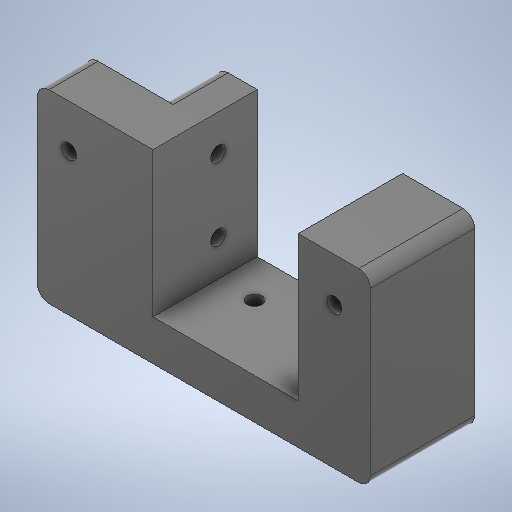
# Autodesk Inventor part: lift_encoder_frame
Saved by Autodesk Inventor 2026.2 (Build 302298010, 298A)
## iProperties
Created: 2026-05-19
Part Number: lift_encoder_frame
Material: ABS Plastic
Document SubType Name: Modeling
Designer: chanh
Density: 1.06 g/cm^3
Appearance: Smooth - White
Author: chanh
Autodesk Inventor part; units mm, degrees
note: some values were not read from the file. Chosen so that the rebuilt part matches the saved one: direction of "Hole3".
ref_plane "YZ Plane" through (0, 0, 0) normal (1, 0, 0) x (0, 1, 0)
ref_plane "XZ Plane" through (0, 0, 0) normal (0, 1, 0) x (-1, 0, 0)
ref_plane "XY Plane" through (0, 0, 0) normal (0, 0, 1) x (1, 0, 0)
sketch "Sketch1" plane through (0, 0, 0) normal (0, 0, 1) x (1, 0, 0)
  line L0 (-50, -64) -> (50, -64)
  line L1 (50, -64) -> (50, 0)
  line L2 (50, 0) -> (-50, 0)
  line L3 (-50, 0) -> (-50, -64)
  line L4 (-50, -64) -> (50, 0) construction
  line L5 (50, -64) -> (-50, 0) construction
  line L6 (-25.1, -50) -> (25.1, -50)
  line L7 (25.1, -50) -> (25.1, 0)
  line L8 (25.1, 0) -> (-25.1, 0)
  line L9 (-25.1, 0) -> (-25.1, -50)
  line L10 (-25.1, -50) -> (25.1, 0) construction
  line L11 (25.1, -50) -> (-25.1, 0) construction
  point P0 (0, 0)
  point P1 (0, -32)
  point P2 (0, 0)
  point P3 (0, -25)
  point P4 (-25.1, 0)
  dimension "d0" = 100
  dimension "d1" = 64
  dimension "d2" = 50.2
  dimension "d3" = 50
  constraints: 24 end point, 6 midpoint, 4 parallel, 2 horizontal, 2 perpendicular, 1 coincident, 1 point on line
  measures "d0" distance of L1.end L2.end
  measures "d1" distance between parallel lines of L2 L0
  measures "d2" distance between parallel lines of L7 L9
  measures "d3" distance between parallel lines of L2 L6
extrude "Extrusion1" add sketch "Sketch1" along normal blind 36 contours L3 L2 L9 L6 L7 L1 L0
sketch "Sketch2" plane through (0, 0, 0) normal (0, 0, -1) x (-1, 0, 0)
  line L0 (-50, 0) -> (-25.1, 0) projected
  line L1 (-25.1, 0) -> (-25.1, -50) projected
  line L2 (-25.1, -50) -> (25.1, -50) projected
  line L3 (25.1, -50) -> (25.1, 0) projected
  line L4 (25.1, 0) -> (50, 0) projected
  line L5 (50, 0) -> (50, -64) projected
  line L6 (50, -64) -> (-50, -64) projected
  line L7 (-50, -64) -> (-50, 0) projected
  line L8 (25.1, 0) -> (50, 0)
  line L9 (50, 0) -> (50, -50)
  line L10 (50, -50) -> (25.1, -50)
  line L11 (25.1, -50) -> (25.1, 0)
  point P0 (0, 0)
  point P1 (25.1, -50)
  constraints: 8 end point, 2 parallel, 1 collinear, 1 horizontal, 1 perpendicular, 1 point on line
extrude "Extrusion2" cut sketch "Sketch2" against normal blind 19 contours L3 L4 L5 L10
sketch "Sketch3" plane through (-50, -64, 0) normal (-1, 0, 0) x (0, 0, 1)
  line L0 (19, 64) -> (19, 14) projected
  line L1 (19, 14) -> (0, 14) projected
  line L2 (0, 14) -> (0, 0) projected
  line L3 (0, 0) -> (36, 0) projected
  line L4 (36, 64) -> (36, 0) projected
  line L5 (19, 64) -> (36, 64) projected
  point P0 (0, 64)
extrude "Extrusion3" add sketch "Sketch3" along normal blind 15
sketch "Sketch4" plane through (0, 0, 0) normal (0, 0, -1) x (-1, 0, 0)
  line L0 (-25.1, -50) -> (65, -50) projected
  line L1 (-25.1, 0) -> (-25.1, -50) projected
  line L2 (-50, 0) -> (-25.1, 0) projected
  line L3 (-50, -64) -> (-50, 0) projected
  line L4 (-50, -64) -> (65, -64) projected
  line L5 (65, -50) -> (65, -64) projected
  line L6 (-50, 0) -> (-25.1, 0) projected
  point P0 (0, 0)
  point P1 (-37.55, -15)
  point P2 (-37.55, 0)
  point P3 (-37.55, 0)
  dimension "d10" = 15
  constraints: 2 midpoint, 1 vertical alignment
  measures "d10" distance of point (-37.55, 0) point (-37.55, -15)
hole "Hole1" at (37.55, -15, 0) direction (0, 0, 1) diameter 5.2 end through all counterbore diameter 10 counterbore depth 14
sketch "Sketch5" plane through (0, 0, 19) normal (0, 0, -1) x (-1, 0, 0)
  line L0 (25.1, 0) -> (65, 0) projected
  line L1 (25.1, -50) -> (25.1, 0) projected
  line L2 (65, -50) -> (25.1, -50) projected
  line L3 (65, 0) -> (65, -50) projected
  line L4 (36.05, -15) -> (54.05, -15) construction
  point P0 (0, 0)
  point P1 (45.05, 0)
  point P2 (45.05, -15)
  dimension "d18" = 18
  dimension "d19" = 15
  constraints: 2 end point, 2 midpoint, 1 horizontal, 1 vertical alignment
  measures "d18" distance of L4.start L4.end
  measures "d19" distance between parallel lines of L4 L0
hole "Hole2" at (-54.05, -15, 19) direction (0, 0, 1) diameter 5.2 end through all counterbore diameter 10 counterbore depth 5
sketch "Sketch6" plane through (0, 0, 19) normal (0, 0, -1) x (-1, 0, 0)
  circle A0 centre (54.05, -15) radius 5 projected
  line L0 (25.1, 0) -> (65, 0) projected
  line L1 (25.1, -50) -> (25.1, 0) projected
  line L2 (65, -50) -> (25.1, -50) projected
  line L3 (65, 0) -> (65, -50) projected
  line L4 (25.1, 0) -> (39.1, 0)
  line L5 (39.1, 0) -> (39.1, -50)
  line L6 (39.1, -50) -> (25.1, -50)
  line L7 (25.1, -50) -> (25.1, 0)
  point P0 (0, 0)
  point P1 (39.1, 0)
  dimension "d27" = 14
  constraints: 8 end point, 2 parallel, 1 horizontal, 1 perpendicular, 1 point on line
  measures "d27" distance between parallel lines of L5 L1
extrude "Extrusion4" add sketch "Sketch6" along normal up to surface (19 mm away) contours L0 L5 L2 L1
sketch "Sketch7" plane through (-39.1, -50, 19) normal (-1, 0, 0) x (0, 0, 1)
  circle A0 centre (-5.5, 37.5) radius 2.067 projected
  circle A1 centre (-5.5, 12.5) radius 2.067 projected
  point P0 (-19, 50)
hole "Hole3" at (-39.1, -12.5, 13.5) at (-39.1, -37.5, 13.5) direction (1, 0, 0) diameter 5.2 depth 14
sketch "Sketch8" plane through (50, -64, 0) normal (0, -1, 0) x (1, 0, 0)
  circle A0 centre (-37.5, 13.5) radius 2.067 projected
  circle A1 centre (-62.5, 13.5) radius 2.067 projected
  point P0 (-50, 0)
hole "Hole4" at (12.5, -64, 13.5) at (-12.5, -64, 13.5) direction (0, 1, 0) diameter 5.2 end through all
fillet "Fillet1" radius 4 7 edges at (50, 0, 18) (50, -64, 18) (-65, -64, 18) (-65, 0, 27.5) (-39.1, -50, 9.5) (-39.1, 0, 9.5) (-65, -50, 9.5)
body "Solid1"
